hexlightsimple (Autodesk Fusion 360 design; units mm, degrees)
Autodesk Fusion 360 part; units mm, degrees
sketch "Sketch1" plane through (0, 0, 0) normal (0, 0, 1) x (1, 0, 0)
  line L0 (86.6025, -50) -> (86.6025, 50)
  line L1 (86.6025, 50) -> (0, 100)
  line L2 (0, 100) -> (-86.6025, 50)
  line L3 (-86.6025, 50) -> (-86.6025, -50)
  line L4 (-86.6025, -50) -> (0, -100)
  line L5 (0, -100) -> (86.6025, -50)
  line L6 (0, -104.6188) -> (90.6025, -52.3094)
  line L7 (90.6025, -52.3094) -> (90.6025, 52.3094)
  line L8 (90.6025, 52.3094) -> (0, 104.6188)
  line L9 (0, 104.6188) -> (-90.6025, 52.3094)
  line L10 (-90.6025, 52.3094) -> (-90.6025, -52.3094)
  line L11 (-90.6025, -52.3094) -> (0, -104.6188)
  line L12 (0, 0) -> (0, -155)
  line L13 (0, -98.8453) -> (85.6025, -49.4226)
  line L14 (85.6025, -49.4226) -> (85.6025, 49.4226)
  line L15 (85.6025, 49.4226) -> (0, 98.8453)
  line L16 (0, 98.8453) -> (-85.6025, 49.4226)
  line L17 (-85.6025, 49.4226) -> (-85.6025, -49.4226)
  line L18 (-85.6025, -49.4226) -> (0, -98.8453)
  line L19 (0, -95.9585) -> (83.1025, -47.9793)
  line L20 (83.1025, -47.9793) -> (83.1025, 47.9793)
  line L21 (83.1025, 47.9793) -> (0, 95.9585)
  line L22 (0, 95.9585) -> (-83.1025, 47.9793)
  line L23 (-83.1025, 47.9793) -> (-83.1025, -47.9793)
  line L24 (-83.1025, -47.9793) -> (0, -95.9585)
  line L25 (-85.6025, -44.4226) -> (-83.1025, -44.4226)
  line L26 (-81.2724, -51.9226) -> (-80.0224, -49.7576)
  line L27 (-56.9017, -65.9931) -> (-55.6517, -63.828)
  line L28 (-28.7008, -82.2749) -> (-27.4508, -80.1098)
  line L29 (-59.9818, -61.328) -> (-61.2318, -63.4931)
  line L30 (-51.3216, -66.328) -> (-52.5716, -68.4931)
  line L31 (-31.781, -77.6098) -> (-33.031, -79.7749)
  line L32 (-23.1207, -82.6098) -> (-24.3707, -84.7749)
  line L33 (-77.8573, -51.0076) -> (-79.1073, -53.1726)
  line L34 (-85.6025, -41.9226) -> (-83.1025, -41.9226)
  line L35 (-40.2522, -72.7189) -> (1.299, -0.75)
  line L36 (1.299, -0.75) -> (-1.299, 0.75)
  line L37 (-1.299, 0.75) -> (-42.8503, -71.2189)
  line L38 (-41.5513, -71.9689) -> (0, 0)
  line L39 (-79.6025, -45.9585) -> (0, -91.9171)
  line L40 (0, -91.9171) -> (79.6025, -45.9585)
  line L41 (79.6025, -45.9585) -> (79.6025, 45.9585)
  line L42 (79.6025, 45.9585) -> (0, 91.9171)
  line L43 (0, 91.9171) -> (-79.6025, 45.9585)
  line L44 (-79.6025, 45.9585) -> (-79.6025, -45.9585)
  line L45 (-45.4304, -65.6878) -> (-47.1804, -68.7189)
  line L46 (-34.1721, -72.1878) -> (-35.9221, -75.2189)
  line L47 (34.1721, -72.1878) -> (35.9221, -75.2189)
  line L48 (45.4304, -65.6878) -> (47.1804, -68.7189)
  line L49 (79.6025, -6.5) -> (83.1025, -6.5)
  line L50 (79.6025, 6.5) -> (83.1025, 6.5)
  line L51 (45.4304, 65.6878) -> (47.1804, 68.7189)
  line L52 (34.1721, 72.1878) -> (35.9221, 75.2189)
  line L53 (-34.1721, 72.1878) -> (-35.9221, 75.2189)
  line L54 (-45.4304, 65.6878) -> (-47.1804, 68.7189)
  line L55 (-79.6025, 6.5) -> (-83.1025, 6.5)
  line L56 (-79.6025, -6.5) -> (-83.1025, -6.5)
  line L57 (0, 90.7624) -> (-78.6025, 45.3812)
  line L58 (-78.6025, 45.3812) -> (-78.6025, -45.3812)
  line L59 (-78.6025, -45.3812) -> (0, -90.7624)
  line L60 (0, -90.7624) -> (78.6025, -45.3812)
  line L61 (78.6025, -45.3812) -> (78.6025, 45.3812)
  line L62 (78.6025, 45.3812) -> (0, 90.7624)
  line L63 (0, -94.5729) -> (81.9025, -47.2865)
  line L64 (81.9025, -47.2865) -> (81.9025, 47.2865)
  line L65 (81.9025, 47.2865) -> (0, 94.5729)
  line L66 (0, 94.5729) -> (-81.9025, 47.2865)
  line L67 (-81.9025, 47.2865) -> (-81.9025, -47.2865)
  line L68 (-81.9025, -47.2865) -> (0, -94.5729)
  dimension "d1" = 100
  dimension "d2" = 4
  dimension "d7" = 1
  dimension "d8" = 2.5
  dimension "d9" = 5
  dimension "d10" = 5
  dimension "d14" = 5
  dimension "d15" = 5
  dimension "d16" = 5
  dimension "d17" = 5
  dimension "d23" = 2.5
  dimension "d155" = 2.5
  dimension "d158" = 3
  dimension "d196" = 16.2818
  dimension "d197" = 16.2818
  dimension "d198" = -3.5
  dimension "d199" = 5
  dimension "d200" = 5
  dimension "d202" = 360
  dimension "d214" = -4.5
  dimension "d215" = -1.2
  constraint coincident L12.start L38.end
  constraint vertical L12
  constraint coincident L4.end L12
  constraint coincident L6.start L12
  constraint coincident L12 L13.start
  constraint coincident L12 L19.start
  constraint coincident L17 L25.start
  constraint coincident L23 L25.end
  constraint perpendicular L23 L25
  constraint coincident L18 L26.start
  constraint coincident L24 L26.end
  constraint perpendicular L24 L26
  constraint coincident L18 L27.start
  constraint coincident L24 L27.end
  constraint perpendicular L24 L27
  constraint coincident L18 L28.start
  constraint coincident L24 L28.end
  constraint perpendicular L24 L28
  constraint coincident L24 L29.start
  constraint coincident L18 L29.end
  constraint perpendicular L18 L29
  constraint coincident L24 L30.start
  constraint coincident L18 L30.end
  constraint perpendicular L18 L30
  constraint coincident L24 L31.start
  constraint coincident L18 L31.end
  constraint perpendicular L18 L31
  constraint coincident L24 L32.start
  constraint coincident L18 L32.end
  constraint perpendicular L18 L32
  constraint coincident L24 L33.start
  constraint coincident L18 L33.end
  constraint perpendicular L18 L33
  constraint coincident L17 L34.start
  constraint coincident L23 L34.end
  constraint perpendicular L23 L34
  constraint coincident L24 L35.start
  constraint perpendicular L24 L35
  constraint perpendicular L35 L36
  constraint coincident L24 L37.end
  constraint perpendicular L24 L37
  constraint midpoint L24 L38.start
  constraint midpoint L36 L12.start
  constraint parallel L35 L38
  constraint coincident L39 L45.start
  constraint coincident L24 L45.end
  constraint perpendicular L24 L45
  constraint coincident L39 L46.start
  constraint coincident L24 L46.end
  constraint perpendicular L24 L46
  measures "d1" distance of L0.start L4.end
  measures "d2" distance of L5 L6
  measures "d7" distance of L5 L13
  measures "d8" distance of L13 L19
  measures "d9" distance of L17.end L25
  measures "d10" distance of L17.end L26
  measures "d14" distance of L28 L32
  measures "d15" distance of L28.end L31.start
  measures "d16" distance of L27.start L30.end
  measures "d17" distance of L27.start L29.end
  measures "d23" distance of L26 L33
  measures "d155" distance of L25 L34
  measures "d158" distance of L35 L37
  measures "d196" distance of L27 L38
  measures "d197" distance of L28 L38
  measures "d199" distance of L35 L46
  measures "d200" distance of L37 L45
extrude "Extrude1" add sketch "Sketch1" against normal blind 2.2 contours L0 L1 L2 L3 L4 L5 | L6 L7 L8 L9 L10 L11 | L12 L37 L39 L40 L41 L42 L43 L44 L57 L58 L59 L60 L61 L62 | L12 L35 L59 | L12 L35 L39 L59 | L12 L35 L36 L37 L57 L58 L59 L60 L61 L62 | L12 L40 L47 L63 | L12 L39 L46 L68 | L12 L35 L38 L59 | L12 L35 L36 | L35 L38 L39 L59 | L12 L19 L47 L63 | L12 L24 L46 L68 | L35 L39 L46 L68 | L40 L47 L48 L63 | L36 L37 L38 L59 | L35 L38 L39 L68 | L37 L38 L39 L59 | L12 L13 L14 L15 L16 L17 L19 L20 L21 L22 L23 L34 | L12 L18 L24 L32 | L19 L47 L48 L63 | L24 L35 L46 L68 | L40 L41 L48 L49 L63 L64 | L24 L35 L38 L68 | L37 L38 L39 L68 | L18 L24 L28 L32 | L19 L20 L48 L49 L63 L64 | L18 L24 L30 L31 | L24 L37 L38 L68 | L37 L39 L45 L68 | L18 L24 L28 L31 | L41 L49 L50 L64 | L24 L37 L45 L68 | L39 L44 L45 L56 L67 L68 | L20 L49 L50 L64 | L41 L42 L50 L51 L64 L65 | L23 L24 L45 L56 L67 L68 | L20 L21 L50 L51 L64 L65 | L18 L24 L27 L30 | L44 L55 L56 L67 | L18 L24 L27 L29 | L42 L51 L52 L65 | L23 L55 L56 L67 | L43 L44 L54 L55 L66 L67 | L17 L23 L25 L34 | L21 L51 L52 L65 | L18 L24 L29 L33 | L42 L43 L52 L53 L65 L66 | L22 L23 L54 L55 L66 L67 | L17 L18 L23 L24 L25 L26 | L21 L22 L52 L53 L65 L66 | L18 L24 L26 L33 | L43 L53 L54 L66 | L22 L53 L54 L66 makes body 1
extrude "Extrude2" add sketch "Sketch1" along normal blind 15 contours L6 L7 L8 L9 L10 L11 bodies 1
extrude "Extrude3" add sketch "Sketch1" along normal blind 9.5 contours L18 L24 L28 L32 | L18 L24 L28 L31 | L18 L24 L27 L30 | L18 L24 L27 L29 | L17 L23 L25 L34 | L18 L24 L26 L33 bodies 1
sketch "Sketch28" plane through (0, 0, 0) normal (0, 0, 1) x (-1, 0, 0)
  line L0 (79.1073, 53.1726) -> (81.2724, 51.9226)
  line L1 (85.6025, 44.4226) -> (85.6025, 41.9226)
  line L2 (-86.6025, 50) -> (-86.6025, -50)
  line L3 (-86.6025, -50) -> (0, -100)
  line L4 (0, -100) -> (86.6025, -50)
  line L5 (86.6025, -50) -> (86.6025, 50)
  line L6 (86.6025, 50) -> (0, 100)
  line L7 (0, 100) -> (-86.6025, 50)
  line L8 (3.0801, 94.1802) -> (-3.0801, 94.1802)
  line L9 (-5.2452, 92.9302) -> (-77.8573, 51.0076)
  line L10 (-80.0224, 49.7576) -> (-83.1025, 44.4226)
  line L11 (-83.1025, 41.9226) -> (-83.1025, -41.9226)
  line L12 (-83.1025, -44.4226) -> (-80.0224, -49.7576)
  line L13 (-77.8573, -51.0076) -> (-5.2452, -92.9302)
  line L14 (-3.0801, -94.1802) -> (3.0801, -94.1802)
  line L15 (5.2452, -92.9302) -> (77.8573, -51.0076)
  line L16 (80.0224, -49.7576) -> (83.1025, -44.4226)
  line L17 (83.1025, -41.9226) -> (83.1025, 41.9226)
  line L18 (83.1025, 44.4226) -> (80.0224, 49.7576)
  line L19 (77.8573, 51.0076) -> (5.2452, 92.9302)
  line L20 (5.2452, 92.9302) -> (3.0801, 94.1802)
  line L21 (-3.0801, 94.1802) -> (-5.2452, 92.9302)
  line L22 (77.8573, 51.0076) -> (80.0224, 49.7576)
  line L23 (83.1025, 44.4226) -> (83.1025, 41.9226)
  line L24 (83.1025, -41.9226) -> (83.1025, -44.4226)
  line L25 (80.0224, -49.7576) -> (77.8573, -51.0076)
  line L26 (5.2452, -92.9302) -> (3.0801, -94.1802)
  line L27 (-3.0801, -94.1802) -> (-5.2452, -92.9302)
  line L28 (-77.8573, -51.0076) -> (-80.0224, -49.7576)
  line L29 (-83.1025, -44.4226) -> (-83.1025, -41.9226)
  line L30 (-83.1025, 41.9226) -> (-83.1025, 44.4226)
  line L31 (-80.0224, 49.7576) -> (-77.8573, 51.0076)
  line L32 (85.6025, 41.9226) -> (83.1025, 41.9226)
  line L33 (83.1025, 41.9226) -> (83.1025, 44.4226)
  line L34 (83.1025, 44.4226) -> (85.6025, 44.4226)
  line L35 (59.9818, 61.328) -> (51.3216, 66.328)
  line L36 (51.3216, 66.328) -> (52.5716, 68.4931)
  line L37 (52.5716, 68.4931) -> (61.2318, 63.4931)
  line L38 (61.2318, 63.4931) -> (59.9818, 61.328)
  line L39 (31.781, 77.6098) -> (23.1207, 82.6098)
  line L40 (23.1207, 82.6098) -> (24.3707, 84.7749)
  line L41 (24.3707, 84.7749) -> (33.031, 79.7749)
  line L42 (33.031, 79.7749) -> (31.781, 77.6098)
  line L43 (81.2724, 51.9226) -> (80.0224, 49.7576)
  line L44 (80.0224, 49.7576) -> (77.8573, 51.0076)
  line L45 (77.8573, 51.0076) -> (79.1073, 53.1726)
extrude "Extrude13" cut sketch "Sketch28" against normal blind 16 contours L8 L9 L10 L11 L12 L13 L14 L15 L16 L17 L18 L19 L20 L21 L22 L23 L24 L25 L26 L27 L28 L29 L30 L31 L33 L35 L39 L44 bodies 1
pattern_circular "C-Pattern11" count 6 over 360 about axis through (0, 0, 1.75) along (0, 0, 1) of "Extrude3"
extrude "Extrude14" add sketch "Sketch1" against normal blind 1.4 contours L12 L35 L38 L59 | L12 L35 L36 | L35 L38 L39 L59 | L36 L37 L38 L59 | L35 L38 L39 L68 | L37 L38 L39 L59 | L24 L35 L38 L68 | L37 L38 L39 L68 | L24 L37 L38 L68 bodies 1
pattern_circular "C-Pattern12" count 6 over 360 about axis through (0, 0, 1.75) along (0, 0, 1) of "Extrude14"
sketch "Sketch29" plane through (0, 0, -1.4) normal (0, 0, -1) x (1, 0, 0)
  line L0 (-83.1025, -44.4226) -> (-83.1025, 44.4226)
  line L1 (-83.1025, 44.4226) -> (-80.0224, 49.7576)
  line L2 (-80.0224, 49.7576) -> (-3.0801, 94.1802)
  line L3 (-42.8503, 71.2189) -> (-2.5981, 1.5)
  line L4 (-2.5981, 1.5) -> (-83.1025, 1.5)
  line L5 (42.8503, -71.2189) -> (2.5981, -1.5)
  line L6 (2.5981, -1.5) -> (83.1025, -1.5)
  line L7 (83.1025, 44.4226) -> (83.1025, -44.4226)
  line L8 (83.1025, -44.4226) -> (80.0224, -49.7576)
  line L9 (80.0224, -49.7576) -> (3.0801, -94.1802)
  line L10 (40.2522, 72.7189) -> (0, 3)
  line L11 (0, 3) -> (-40.2522, 72.7189)
  line L12 (-3.0801, 94.1802) -> (3.0801, 94.1802)
  line L13 (3.0801, 94.1802) -> (80.0224, 49.7576)
  line L14 (0, 104.6188) -> (-90.6025, 52.3094)
  line L15 (-90.6025, 52.3094) -> (-90.6025, -52.3094)
  line L16 (-90.6025, -52.3094) -> (0, -104.6188)
  line L17 (0, -104.6188) -> (90.6025, -52.3094)
  line L18 (90.6025, -52.3094) -> (90.6025, 52.3094)
  line L19 (90.6025, 52.3094) -> (0, 104.6188)
  line L20 (83.1025, 1.5) -> (2.5981, 1.5)
  line L21 (2.5981, 1.5) -> (42.8503, 71.2189)
  line L22 (80.0224, 49.7576) -> (83.1025, 44.4226)
  line L23 (83.1025, -1.5) -> (83.1025, 1.5)
  line L24 (-40.2522, -72.7189) -> (0, -3)
  line L25 (0, -3) -> (40.2522, -72.7189)
  line L26 (3.0801, -94.1802) -> (-3.0801, -94.1802)
  line L27 (-3.0801, -94.1802) -> (-80.0224, -49.7576)
  line L28 (-83.1025, -1.5) -> (-2.5981, -1.5)
  line L29 (-2.5981, -1.5) -> (-42.8503, -71.2189)
  line L30 (-80.0224, -49.7576) -> (-83.1025, -44.4226)
  line L31 (-83.1025, 1.5) -> (-83.1025, -1.5)
  line L32 (-3.0801, 94.1802) -> (-40.2522, 72.7189)
  line L33 (-40.2522, 72.7189) -> (0, 3)
  line L34 (-3.0801, 94.1802) -> (3.0801, 94.1802)
  line L35 (3.0801, 94.1802) -> (80.0224, 49.7576)
  line L36 (80.0224, 49.7576) -> (0, 3)
  line L37 (-3.0801, 94.1802) -> (-80.0224, 49.7576)
  line L38 (-80.0224, 49.7576) -> (-83.1025, 44.4226)
  line L39 (-83.1025, 44.4226) -> (-83.1025, -44.4226)
  line L40 (-83.1025, -44.4226) -> (-80.0224, -49.7576)
  line L41 (-80.0224, -49.7576) -> (-3.0801, -94.1802)
  line L42 (-3.0801, -94.1802) -> (3.0801, -94.1802)
  line L43 (3.0801, -94.1802) -> (80.0224, -49.7576)
  line L44 (80.0224, -49.7576) -> (83.1025, -44.4226)
  line L45 (83.1025, -44.4226) -> (83.1025, 44.4226)
  line L46 (83.1025, 44.4226) -> (80.0224, 49.7576)
  line L47 (80.0224, 49.7576) -> (3.0801, 94.1802)
  line L48 (-40.2522, 72.7189) -> (-39.3888, 71.2234)
  line L49 (-35.0381, 71.6878) -> (-36.7881, 74.7189)
  line L50 (-46.3144, 69.2189) -> (-44.5644, 66.1878)
  line L51 (-41.5513, 71.9689) -> (0, 0)
  line L52 (-1.3301, 91.1491) -> (-77.4602, 47.1954)
  line L53 (-77.4602, 47.1954) -> (-79.6025, 43.4848)
  line L54 (-79.6025, 43.4848) -> (-79.6025, -43.4848)
  line L55 (-79.6025, -43.4848) -> (-77.4602, -47.1954)
  line L56 (-77.4602, -47.1954) -> (-2.1423, -90.6802)
  line L57 (-2.1423, -90.6802) -> (2.1423, -90.6802)
  line L58 (2.1423, -90.6802) -> (77.4602, -47.1954)
  line L59 (77.4602, -47.1954) -> (79.6025, -43.4848)
  line L60 (79.6025, -43.4848) -> (79.6025, 43.4848)
  line L61 (79.6025, 43.4848) -> (77.4602, 47.1954)
  line L62 (77.4602, 47.1954) -> (1.3301, 91.1491)
  line L63 (-79.6025, 45.9585) -> (0, 91.9171)
  line L64 (-42.8503, -71.2189) -> (-40.2522, -72.7189)
  line L65 (40.2522, -72.7189) -> (42.8503, -71.2189)
  line L66 (42.8503, 71.2189) -> (40.2522, 72.7189)
  line L67 (-40.2522, 72.7189) -> (-42.8503, 71.2189)
  line L68 (-79.6025, 43.4848) -> (-79.6025, -43.4848)
  line L69 (-79.6025, -43.4848) -> (-77.4602, -47.1954)
  line L70 (-77.4602, -47.1954) -> (-2.1423, -90.6802)
  line L71 (-2.1423, -90.6802) -> (2.1423, -90.6802)
  line L72 (2.1423, -90.6802) -> (77.4602, -47.1954)
  line L73 (77.4602, -47.1954) -> (79.6025, -43.4848)
  line L74 (79.6025, -43.4848) -> (79.6025, 43.4848)
  line L75 (79.6025, 43.4848) -> (77.4602, 47.1954)
  line L76 (77.4602, 47.1954) -> (2.1423, 90.6802)
  line L77 (-2.1423, 90.6802) -> (2.1423, 90.6802)
  line L78 (-2.1423, 90.6802) -> (-77.4602, 47.1954)
  line L79 (-77.4602, 47.1954) -> (-79.6025, 43.4848)
  dimension "d209" = 5.5
  dimension "d210" = 5.5
  dimension "d211" = -3.5
  dimension "d222" = -3.5
  constraint coincident L2.end L12.start
  constraint coincident L11.end L32.end
  constraint coincident L10.end L11.start
  constraint coincident L12.end L13.start
  constraint coincident L13.end L22.start
  constraint coincident L1.end L2.start
  constraint coincident L0.end L1.start
  constraint coincident L0.start L30.end
  constraint coincident L27.end L30.start
  constraint coincident L26.end L27.start
  constraint coincident L9.end L26.start
  constraint coincident L8.end L9.start
  constraint coincident L7.end L8.start
  constraint coincident L7.start L22.end
  constraint coincident L33 L48.end
  constraint coincident L37 L49.end
  constraint coincident L2 L50.start
  constraint coincident L49.start L63
  constraint coincident L50.end L63
  measures "d209" distance of L50 L51
  measures "d210" distance of L49 L51
extrude "Extrude1'" add sketch "Sketch29" along normal blind 5 from surface at 0.8 separate body contours L0 L27 L28 L29 L30 L39 L40 L41 L54 L55 L56 L68 L69 L70 | L0 L4 L28 L31 L39 L54 L68 | L0 L1 L2 L4 L37 L38 L39 L50 L52 L53 L54 L63 L68 L78 L79 | L24 L27 L29 L41 L56 L64 L70 | L9 L24 L25 L26 L27 L41 L42 L43 L56 L57 L58 L70 L71 L72 | L2 L3 L37 L50 L52 L63 L78 | L2 L3 L37 L51 L52 L63 L67 L78 | L2 L11 L33 L37 L48 L51 L52 L63 L67 L78 | L5 L9 L25 L43 L58 L65 L72 | L2 L11 L32 L33 L37 L48 L49 L52 L63 L78 | L5 L6 L7 L8 L9 L43 L44 L45 L58 L59 L60 L72 L73 L74 | L2 L10 L12 L13 L32 L34 L35 L37 L47 L49 L52 L62 L63 L76 L77 L78 | L10 L13 L21 L35 L47 L62 L66 L76 | L6 L7 L20 L23 L45 L60 L74 | L13 L21 L35 L36 L47 L62 L76 | L7 L20 L22 L36 L45 L46 L60 L61 L62 L74 L75 L76 makes body 2 in component "Back "
extrude "Extrude16" add sketch "Sketch1" against normal blind 2.2 separate body contours L35 L39 L46 L68 | L35 L38 L39 L68 | L24 L35 L46 L68 | L24 L35 L38 L68 | L37 L38 L39 L68 | L24 L37 L38 L68 | L37 L39 L45 L68 | L24 L37 L45 L68 makes body 3
sketch "Sketch30" plane through (0, 0, 15) normal (0, 0, 1) x (-1, 0, 0)
  line L0 (-86.6025, 50) -> (0, 100)
  line L1 (0, 100) -> (86.6025, 50)
  line L2 (86.6025, 50) -> (86.6025, -50)
  line L3 (86.6025, -50) -> (0, -100)
  line L4 (0, -100) -> (-86.6025, -50)
  line L5 (-86.6025, -50) -> (-86.6025, 50)
  line L6 (90.6025, 52.3094) -> (0, 104.6188)
  line L7 (0, 104.6188) -> (-90.6025, 52.3094)
  line L8 (-90.6025, 52.3094) -> (-90.6025, -52.3094)
  line L9 (-90.6025, -52.3094) -> (0, -104.6188)
  line L10 (0, -104.6188) -> (90.6025, -52.3094)
  line L11 (90.6025, -52.3094) -> (90.6025, 52.3094)
  line L12 (0, -100) -> (86.6025, -50)
  line L13 (86.6025, 50) -> (86.6025, -50)
  line L14 (86.6025, 50) -> (0, 100)
  line L15 (0, 100) -> (-86.6025, 50)
  line L16 (-86.6025, 50) -> (-86.6025, -50)
  line L17 (-86.6025, -50) -> (0, -100)
  constraint coincident L3.end L4.start
  constraint coincident L2.end L3.start
  constraint coincident L1.end L2.start
  constraint coincident L0.end L1.start
  constraint coincident L0.start L5.end
  constraint coincident L4.end L5.start
extrude "Extrude1''" add sketch "Sketch30" against normal blind 3 separate body contours L0 L1 L2 L3 L4 L5 L12 L13 L14 L15 L16 L17 makes body 4 in component "Top"
sketch "Sketch32" plane through (0, 0, 12) normal (0, 0, -1) x (1, 0, 0)
  line L0 (0, 100) -> (-86.6025, 50)
  line L1 (-86.6025, 50) -> (-86.6025, -50)
  line L2 (-86.6025, -50) -> (0, -100)
  line L3 (0, -100) -> (86.6025, -50)
  line L4 (86.6025, -50) -> (86.6025, 50)
  line L5 (86.6025, 50) -> (0, 100)
  line L6 (-86.6025, -20.8333) -> (-83.1025, -20.8333)
  line L7 (-83.1025, -20.8333) -> (-83.1025, -12.8333)
  line L8 (-83.1025, -12.8333) -> (-86.6025, -12.8333)
  line L9 (-86.6025, -12.8333) -> (-86.6025, -20.8333)
  line L10 (-86.6025, 12.8333) -> (-83.1025, 12.8333)
  line L11 (-83.1025, 12.8333) -> (-83.1025, 20.8333)
  line L12 (-83.1025, 20.8333) -> (-86.6025, 20.8333)
  line L13 (-86.6025, 20.8333) -> (-86.6025, 12.8333)
  line L14 (-86.6025, 20.8333) -> (-86.6025, 12.8333)
  line L15 (-86.6025, 50) -> (-86.6025, -50)
  line L16 (-86.6025, -12.8333) -> (-86.6025, -20.8333)
  line L17 (-86.2025, -12.8333) -> (-86.2025, -20.8333)
  line L18 (-86.2025, 20.8333) -> (-86.2025, 12.8333)
  dimension "d180" = 3.5
  dimension "d181" = 3.5
  dimension "d182" = 8
  dimension "d183" = 8
  dimension "d187" = 100
  dimension "d188" = 29.1667
  dimension "d189" = 29.1667
  dimension "d190" = -0.4
  dimension "d191" = -0.4
  constraint horizontal L6
  constraint vertical L7
  constraint horizontal L8
  constraint vertical L9
  constraint coincident L1 L6.start
  constraint horizontal L10
  constraint vertical L11
  constraint horizontal L12
  constraint vertical L13
  constraint coincident L1 L10.start
  constraint coincident L0.end L1.start
  constraint coincident L1.end L2.start
  measures "d180" distance of L6.start L6.end
  measures "d181" distance of L10.start L10.end
  measures "d182" distance of L6.end L7.end
  measures "d183" distance of L10.end L11.end
  measures "d187" distance of L0.end L1.end
  measures "d188" distance of L6 L1.end
  measures "d189" distance of L12 L0.end
extrude "Extrude18" add sketch "Sketch32" along normal blind 2.5 separate body contours L10 L11 L12 L18 | L6 L7 L8 L17 makes body 5 at (-85.1692, -18.1667, 12) makes body 6 at (-85.1692, 18.1667, 12)
pattern_circular "C-Pattern13" count 6 over 360 about axis through (0, 0, 1.75) along (0, 0, 1) of "Extrude18" makes body 7 at (-26.8518, -82.842, 12) makes body 8 at (-58.3174, -64.6754, 12) makes body 9 at (55.4913, -65.1138, 12) makes body 10 at (26.3351, -81.9471, 12) makes body 11 at (85.1692, 18.1667, 12) makes body 12 at (85.1692, -18.1667, 12) makes body 13 at (29.1612, 81.5087, 12) makes body 14 at (57.8007, 63.7805, 12) makes body 15 at (-56.008, 66.0087, 12) makes body 16 at (-26.8518, 82.842, 12)
copy_body "CutPasteBodies1" bodies 5 6 7 8 9 10 11 12 13 14 15 16 removing the originals makes body 17 makes body 18 makes body 19 makes body 20 makes body 21 makes body 22 makes body 23 makes body 24 makes body 25 makes body 26 makes body 27 makes body 28 in component "Top"
combine "Combine1" operation add target body 4 tool bodies 24 25 21 17 23 26 28 27 20 18 19 22 in component "Top"
extrude "Extrude19" add sketch "Sketch1" against normal blind 1.4 contours L12 L40 L47 L63 | L12 L39 L46 L68 | L12 L19 L47 L63 | L12 L24 L46 L68 | L40 L41 L48 L49 L63 L64 | L19 L20 L48 L49 L63 L64 | L39 L44 L45 L56 L67 L68 | L41 L42 L50 L51 L64 L65 | L23 L24 L45 L56 L67 L68 | L20 L21 L50 L51 L64 L65 | L43 L44 L54 L55 L66 L67 | L42 L43 L52 L53 L65 L66 | L22 L23 L54 L55 L66 L67 | L21 L22 L52 L53 L65 L66 bodies 1
extrude "Extrude20" cut sketch "Sketch1" against normal blind 1.4 contours L12 L35 L38 L59 | L12 L35 L36 | L35 L38 L39 L59 | L36 L37 L38 L59 | L35 L38 L39 L68 | L37 L38 L39 L59 | L24 L35 L38 L68 | L37 L38 L39 L68 | L24 L37 L38 L68 bodies 1
pattern_circular "C-Pattern14" count 6 over 360 about axis through (0, 0, 1.75) along (0, 0, 1) of "Extrude20"
copy_body "CutPasteBodies2" bodies 3 removing the originals makes body 29 in component "Back "
pattern_circular "C-Pattern2" count 6 over 360 about axis through (0, 0, 1.75) along (0, 0, 1) of bodies 29 makes body 30 at (38.0255, -72.1955, 0) makes body 31 at (81.5359, -3.1667, 0) makes body 32 at (43.5104, 69.0288, 0) makes body 33 at (-38.0255, 72.1955, 0) makes body 34 at (-81.5359, 3.1667, 0) in component "Back "
combine "Combine2" operation add target body 2 tool bodies 29 31 30 32 33 34 in component "Back "
extrude "Extrude22" add sketch "Sketch1" against normal blind 2.2 contours L12 L37 L39 L40 L41 L42 L43 L44 L57 L58 L59 L60 L61 L62 | L12 L35 L39 L59 | L12 L40 L47 L63 | L12 L39 L46 L68 | L35 L38 L39 L59 | L12 L19 L47 L63 | L12 L24 L46 L68 | L37 L38 L39 L59 | L40 L41 L48 L49 L63 L64 | L19 L20 L48 L49 L63 L64 | L39 L44 L45 L56 L67 L68 | L41 L42 L50 L51 L64 L65 | L23 L24 L45 L56 L67 L68 | L20 L21 L50 L51 L64 L65 | L43 L44 L54 L55 L66 L67 | L42 L43 L52 L53 L65 L66 | L22 L23 L54 L55 L66 L67 | L21 L22 L52 L53 L65 L66 bodies 1
extrude "Extrude23" cut sketch "Sketch1" against normal blind 2 contours L12 L40 L47 L63 | L12 L39 L46 L68 | L35 L39 L46 L68 | L40 L47 L48 L63 | L35 L38 L39 L68 | L40 L41 L48 L49 L63 L64 | L37 L38 L39 L68 | L37 L39 L45 L68 | L41 L49 L50 L64 | L39 L44 L45 L56 L67 L68 | L41 L42 L50 L51 L64 L65 | L44 L55 L56 L67 | L42 L51 L52 L65 | L43 L44 L54 L55 L66 L67 | L42 L43 L52 L53 L65 L66 | L43 L53 L54 L66 bodies 1
extrude "Extrude2'" cut sketch "Sketch1" against normal blind 2 contours L12 L40 L47 L63 | L12 L39 L46 L68 | L35 L39 L46 L68 | L40 L47 L48 L63 | L35 L38 L39 L68 | L40 L41 L48 L49 L63 L64 | L37 L38 L39 L68 | L37 L39 L45 L68 | L41 L49 L50 L64 | L39 L44 L45 L56 L67 L68 | L41 L42 L50 L51 L64 L65 | L44 L55 L56 L67 | L42 L51 L52 L65 | L43 L44 L54 L55 L66 L67 | L42 L43 L52 L53 L65 L66 | L43 L53 L54 L66 bodies 2 in component "Back "
component "Back " placed x (1, 0, 0) y (0, 1, 0) z (0, 0, 1) at (0, 0, 0)
component "Top" placed x (1, 0, 0) y (0, 1, 0) z (0, 0, 1) at (0, 0, 0)
equation "d9 = d10"
equation "d14 = d17"
equation "d15 = d17"
equation "d16 = d17"
equation "d22 = d9 / 2"
equation "d23 = d155"
equation "d27 = d22 - d8"
equation "d181 = d180"
equation "d183 = d182"
equation "d188 = ( ( ( 100.00 / 2 ) * 1 mm ) / 3 ) * 1.75"
equation "d189 = d188"
equation "d197 = d196"
equation "d200 = d199"
equation "d210 = d209"
